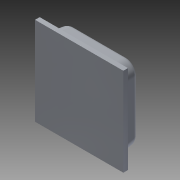
# Autodesk Inventor part: BMP180
Saved by Autodesk Inventor 2013 (Build 170138000, 138)
## iProperties
Created: 2015-06-30
Part Number: BMP180
Material: Ogólny
Document SubType Name: Modeling
Designer: terg
Density: 1 g/cm^3
Author: terg
Autodesk Inventor part; units mm, degrees
ref_plane "YZ Plane" through (0, 0, 0) normal (1, 0, 0) x (0, 1, 0)
ref_plane "XZ Plane" through (0, 0, 0) normal (0, 1, 0) x (-1, 0, 0)
sketch "Szkic1" plane through (0, 0, 0) normal (0, 1, 0) x (-1, 0, 0)
  line L0 (0, 0) -> (3.8, 0)
  line L1 (3.8, 0) -> (3.8, 3.8)
  line L2 (3.8, 3.8) -> (0, 3.8)
  line L3 (0, 3.8) -> (0, 0)
  dimension "d0" = 3.8
  dimension "d1" = 3.8
  constraints: 8 end point, 2 parallel, 1 horizontal, 1 perpendicular
  measures "d0" distance of L2.end L1.end
  measures "d1" distance of L1.end L0.end
extrude "Wyciągnięcie proste1" add sketch "Szkic1" along normal blind 0.2
sketch "Szkic2" plane through (0, 0.2, 0) normal (0, 1, 0) x (1, 0, 0)
  line L0 (0, 0) -> (-3.8, 0) projected
  line L1 (-3.8, 0) -> (-3.8, -3.8) projected
  line L2 (-3.8, -3.8) -> (0, -3.8) projected
  line L3 (0, -3.8) -> (0, 0) projected
  line L4 (-3.075, -0.225) -> (-0.725, -0.225)
  line L5 (-0.225, -0.725) -> (-0.225, -3.075)
  line L6 (-0.725, -3.575) -> (-3.075, -3.575)
  line L7 (-3.575, -3.075) -> (-3.575, -0.725)
  arc A0 (-3.075, -0.225) -> (-3.575, -0.725) centre (-3.075, -0.725) ccw
  arc A1 (-0.225, -0.725) -> (-0.725, -0.225) centre (-0.725, -0.725) ccw
  arc A2 (-0.725, -3.575) -> (-0.225, -3.075) centre (-0.725, -3.075) ccw
  arc A3 (-3.575, -3.075) -> (-3.075, -3.575) centre (-3.075, -3.075) ccw
  point P0 (-0.225, -3.575)
  point P1 (-0.225, -0.225)
  point P2 (-3.575, -3.575)
  dimension "d4" = 3.35
  dimension "d5" = 3.35
  dimension "d6" = 0.225
  dimension "d7" = 0.225
  dimension "d8" = 0.225
  dimension "d9" = 0.225
  dimension "d10" = 0.5
  constraints: 8 end point, 8 point on circle, 8 tangent, 6 point on line, 4 centre point, 3 equal radius, 2 parallel, 1 horizontal, 1 perpendicular
  measures "d4" distance of point (-0.225, -3.575) point (-3.575, -3.575)
  measures "d5" distance of point (-0.225, -0.225) point (-0.225, -3.575)
  measures "d6" distance between parallel lines of L0 L4
  measures "d7" distance between parallel lines of L2 L6
  measures "d8" distance between parallel lines of L3 L5
  measures "d9" distance between parallel lines of L1 L7
  measures "d10" radius of A0
ref_plane "Płaszczyzna konstrukcyjna1" through (0, 0.93, 0) normal (0, 1, 0) x (1, 0, 0)
sketch "Szkic3" plane through (0, 0.93, 0) normal (0, 1, 0) x (1, 0, 0)
  line L0 (-3, -0.3) -> (-0.8, -0.3)
  line L1 (-0.3, -0.8) -> (-0.3, -3)
  line L2 (-0.8, -3.5) -> (-3, -3.5)
  line L3 (-3.5, -3) -> (-3.5, -0.8)
  line L4 (-3.8, -3.8) -> (0, -3.8) projected
  line L5 (0, 0) -> (-3.8, 0) projected
  line L6 (-3.8, 0) -> (-3.8, -3.8) projected
  line L7 (0, -3.8) -> (0, 0) projected
  arc A0 (-3, -0.3) -> (-3.5, -0.8) centre (-3, -0.8) ccw
  arc A1 (-0.3, -0.8) -> (-0.8, -0.3) centre (-0.8, -0.8) ccw
  arc A2 (-0.8, -3.5) -> (-0.3, -3) centre (-0.8, -3) ccw
  arc A3 (-3.5, -3) -> (-3, -3.5) centre (-3, -3) ccw
  point P0 (-0.3, -3.5)
  point P1 (-0.3, -0.3)
  point P2 (-3.5, -3.5)
  dimension "d12" = 3.2
  dimension "d13" = 3.2
  dimension "d14" = 0.3
  dimension "d15" = 0.3
  dimension "d16" = 0.3
  dimension "d17" = 0.3
  dimension "d18" = 0.5
  constraints: 8 end point, 8 point on circle, 8 tangent, 6 point on line, 4 centre point, 3 equal radius, 2 parallel, 1 horizontal, 1 perpendicular
  measures "d12" distance of point (-0.3, -3.5) point (-3.5, -3.5)
  measures "d13" distance of point (-0.3, -0.3) point (-0.3, -3.5)
  measures "d14" distance between parallel lines of L4 L2
  measures "d15" distance between parallel lines of L5 L0
  measures "d16" distance between parallel lines of L6 L3
  measures "d17" distance between parallel lines of L7 L1
  measures "d18" radius of A0
loft "Wyciągnięcie złożone1" add profiles "Szkic2", "Szkic3" contours L4 A1 L5 A2 L6 A3 L7 A0 / L0 A1 L1 A2 L2 A3 L3 A0
sketch "Szkic4" plane through (-3, 0.93, 0.3) normal (0, 1, 0) x (1, 0, 0)
  point P0 (3, 0.3)
  point P1 (1.775, -0.55)
  dimension "d23" = 1.225
  dimension "d24" = 0.85
  measures "d23" horizontal distance of point (3, 0.3) point (1.775, -0.55)
  measures "d24" vertical distance of point (3, 0.3) point (1.775, -0.55)
hole "Otwór1" at (-1.225, 0.93, 0.85) direction (0, -1, 0) diameter 0.5 depth 0.1
sketch "Szkic5" plane through (-3, 0.93, 0.3) normal (0, 1, 0) x (1, 0, 0)
  line L0 (0.069, -2.9033) -> (0.657, -2.9033)
  line L1 (0.657, -2.9033) -> (0.657, -2.8361)
  line L2 (0.657, -2.8361) -> (0.069, -2.8361)
  line L3 (0.069, -2.8361) -> (0.069, -2.9033)
  line L4 (0.069, -2.8361) -> (0.1501, -2.8361)
  line L5 (0.1501, -2.8361) -> (0.1501, -2.5827)
  line L6 (0.1501, -2.5827) -> (0.069, -2.5827)
  line L7 (0.069, -2.5827) -> (0.069, -2.8361)
  line L8 (0.363, -2.8361) -> (0.292, -2.8361)
  line L9 (0.292, -2.8361) -> (0.292, -2.5827)
  line L10 (0.292, -2.5827) -> (0.363, -2.5827)
  line L11 (0.363, -2.5827) -> (0.363, -2.8361)
  line L12 (0.5759, -2.8361) -> (0.657, -2.8361)
  line L13 (0.657, -2.8361) -> (0.657, -2.5827)
  line L14 (0.657, -2.5827) -> (0.5759, -2.5827)
  line L15 (0.5759, -2.5827) -> (0.5759, -2.8361)
  line L16 (0.363, -2.5827) -> (0.6165, -2.5827)
  line L17 (0.6165, -2.5827) -> (0.6165, -2.518)
  line L18 (0.6165, -2.518) -> (0.363, -2.518)
  line L19 (0.363, -2.518) -> (0.363, -2.5827)
  line L20 (0.1095, -2.5827) -> (0.3275, -2.5827)
  line L21 (0.3275, -2.5827) -> (0.3275, -2.518)
  line L22 (0.3275, -2.518) -> (0.1095, -2.518)
  line L23 (0.1095, -2.518) -> (0.1095, -2.5827)
  line L24 (0.069, -2.3829) -> (0.657, -2.3829)
  line L25 (0.657, -2.3829) -> (0.657, -2.3101)
  line L26 (0.657, -2.3101) -> (0.069, -2.3101)
  line L27 (0.069, -2.3101) -> (0.069, -2.3829)
  line L28 (0.069, -2.3829) -> (0.4897, -2.1887)
  line L29 (0.4897, -2.1887) -> (0.4897, -2.0923)
  line L30 (0.4897, -2.0923) -> (0.0622, -1.9179)
  line L31 (0.0622, -1.9179) -> (0.657, -1.9179)
  line L32 (0.657, -1.9179) -> (0.657, -1.9902)
  line L33 (0.657, -1.9902) -> (0.0622, -1.9902)
  line L34 (0.0622, -1.9902) -> (0.0622, -1.9179)
  line L35 (0.069, -2.3101) -> (0.3833, -2.165)
  line L36 (0.3833, -2.165) -> (0.3833, -2.1212)
  line L37 (0.3833, -2.1212) -> (0.0622, -1.9902)
  line L38 (0.0622, -1.7847) -> (0.657, -1.7847)
  line L39 (0.657, -1.7847) -> (0.657, -1.7194)
  line L40 (0.657, -1.7194) -> (0.0622, -1.7194)
  line L41 (0.0622, -1.7194) -> (0.0622, -1.7847)
  line L42 (0.0622, -1.7194) -> (0.1253, -1.7194)
  line L43 (0.1253, -1.7194) -> (0.1253, -1.4987)
  line L44 (0.1253, -1.4987) -> (0.0622, -1.4987)
  line L45 (0.0622, -1.4987) -> (0.0622, -1.7194)
  line L46 (0.2794, -1.7194) -> (0.3275, -1.7194)
  line L47 (0.3275, -1.7194) -> (0.3275, -1.4987)
  line L48 (0.3275, -1.4987) -> (0.2794, -1.4987)
  line L49 (0.2794, -1.4987) -> (0.2794, -1.7194)
  line L50 (0.0938, -1.4987) -> (0.3034, -1.4987)
  line L51 (0.3034, -1.4987) -> (0.3034, -1.4492)
  line L52 (0.3034, -1.4492) -> (0.0938, -1.4492)
  line L53 (0.0938, -1.4492) -> (0.0938, -1.4987)
  line L54 (0.0724, -1.3337) -> (0.6671, -1.3337)
  line L55 (0.6671, -1.3337) -> (0.6671, -1.246)
  line L56 (0.6671, -1.246) -> (0.0724, -1.246)
  line L57 (0.0724, -1.246) -> (0.0724, -1.3337)
  line L58 (0.0724, -1.1182) -> (0.6671, -1.1182)
  line L59 (0.6671, -1.1182) -> (0.6671, -1.0396)
  line L60 (0.6671, -1.0396) -> (0.0724, -1.0396)
  line L61 (0.0724, -1.0396) -> (0.0724, -1.1182)
  line L62 (0.0724, -0.8686) -> (0.6671, -0.8686)
  line L63 (0.6671, -0.8686) -> (0.6671, -0.7845)
  line L64 (0.6671, -0.7845) -> (0.0724, -0.7845)
  line L65 (0.0724, -0.7845) -> (0.0724, -0.8686)
  line L66 (0.0724, -1.1182) -> (0.1354, -1.1182)
  line L67 (0.1354, -1.1182) -> (0.1354, -0.7845)
  line L68 (0.1354, -0.7845) -> (0.0724, -0.7845)
  line L69 (0.0724, -0.7845) -> (0.0724, -1.1182)
  line L70 (0.6006, -1.1182) -> (0.6671, -1.1182)
  line L71 (0.6671, -1.1182) -> (0.6671, -0.7845)
  line L72 (0.6671, -0.7845) -> (0.6006, -0.7845)
  line L73 (0.6006, -0.7845) -> (0.6006, -1.1182)
  line L74 (0.3136, -1.1182) -> (0.3934, -1.1182)
  line L75 (0.3934, -1.1182) -> (0.3934, -0.7845)
  line L76 (0.3934, -0.7845) -> (0.3136, -0.7845)
  line L77 (0.3136, -0.7845) -> (0.3136, -1.1182)
  line L78 (0.0724, -0.6598) -> (0.6671, -0.6598)
  line L79 (0.6671, -0.6598) -> (0.6671, -0.6028)
  line L80 (0.6671, -0.6028) -> (0.0724, -0.6028)
  line L81 (0.0724, -0.6028) -> (0.0724, -0.6598)
  line L82 (0.0724, -0.6598) -> (0.1354, -0.6598)
  line L83 (0.1354, -0.6598) -> (0.1354, -0.3885)
  line L84 (0.1354, -0.3885) -> (0.0724, -0.3885)
  line L85 (0.0724, -0.3885) -> (0.0724, -0.6598)
  line L86 (0.6006, -0.6598) -> (0.6671, -0.6598)
  line L87 (0.6671, -0.6598) -> (0.6671, -0.3885)
  line L88 (0.6671, -0.3885) -> (0.6006, -0.3885)
  line L89 (0.6006, -0.3885) -> (0.6006, -0.6598)
  line L90 (0.0724, -0.3885) -> (0.6671, -0.3885)
  line L91 (0.6671, -0.3885) -> (0.6671, -0.3261)
  line L92 (0.6671, -0.3261) -> (0.0724, -0.3261)
  line L93 (0.0724, -0.3261) -> (0.0724, -0.3885)
  point P0 (3, 0.3)
  constraints: 188 end point, 46 parallel, 25 perpendicular, 21 horizontal, 7 point on line, 3 midpoint
extrude "Wyciągnięcie proste2" cut sketch "Szkic5" against normal blind 0.05 contours L3 L2 L1 L0 | L7 L6 L5 L2 | L2 L15 L14 L13 | L9 L10 L11 L2 | L6 L23 L22 L21 L10 L20 | L16 L19 L18 L17 L14 | L28 L26 L25 L24 | L27 L26 L28 | L35 L36 L37 L33 L30 L29 L28 L26 | L34 L30 L33 | L30 L31 L32 L33 | L41 L40 L39 L38 | L45 L44 L43 L40 | L40 L49 L48 L47 | L44 L53 L52 L51 L48 L50 | L57 L56 L55 L54 | L61 L60 L67 L58 | L67 L60 L77 L58 | L69 L62 L67 L60 | L77 L60 L75 L58 | L65 L64 L67 L62 | L75 L60 L73 L58 | L77 L62 L75 L60 | L67 L64 L77 L62 | L73 L60 L59 L58 | L77 L64 L75 L62 | L73 L62 L71 L60 | L75 L64 L73 L62 | L73 L64 L63 L62 | L81 L80 L83 L78 | L83 L80 L89 L78 | L85 L84 L83 L80 | L89 L80 L79 L78 | L93 L92 L91 L88 L90 L84 | L89 L88 L87 L80
fillet "Zaokrąglenie1" radius 0.2 8 edges at (-3.3536, 0.93, 3.3536) (-3.5, 0.93, 1.9) (-3.3536, 0.93, 0.4464) (-1.9, 0.93, 0.3) (-0.4464, 0.93, 0.4464) (-0.3, 0.93, 1.9) (-0.4464, 0.93, 3.3536) (-1.9, 0.93, 3.5)
equation "\"d6\" = d7"
equation "\"d8\" = d9"
equation "\"d14\" = d15"
equation "\"d16\" = d17"
